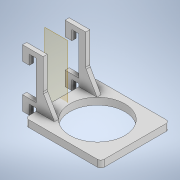
# Autodesk Inventor part: round_2_0_inchHoleV01
Saved by Autodesk Inventor 2021 (Build 250183000, 183)
## iProperties
Created: 2020-03-07
Part Number: round_2_0_inchHoleV01
Material: Generic
Document SubType Name: Modeling
Designer: robst
Density: 1 g/cm^3
Appearance: Default
Author: robst
Autodesk Inventor part; units mm, degrees
ref_plane "YZ Plane" through (0, 0, 0) normal (1, 0, 0) x (0, 1, 0)
ref_plane "XZ Plane" through (0, 0, 0) normal (0, 1, 0) x (-1, 0, 0)
sketch "Sketch1" plane through (0, 0, 0) normal (0, 0, 1) x (1, 0, 0)
  line L0 (0, 6.35) -> (0, 53.34)
  line L1 (0, 53.34) -> (-19.05, 53.34)
  line L2 (-19.05, 53.34) -> (-19.05, 55.245)
  line L3 (-12.7, 48.895) -> (-6.35, 48.895)
  line L4 (-6.35, 48.895) -> (-6.35, 13.335)
  line L5 (-6.35, 13.335) -> (-19.05, 13.335)
  line L6 (-19.05, 13.335) -> (-19.05, 12.7)
  line L7 (-12.7, 8.89) -> (-6.35, 8.89)
  line L8 (-6.35, 8.89) -> (-6.35, 0)
  line L9 (-6.35, 0) -> (0, 0)
  line L10 (-19.05, 55.245) -> (-19.05, 40.005)
  line L11 (-19.05, 40.005) -> (-12.7, 40.005)
  line L12 (-12.7, 40.005) -> (-12.7, 48.895)
  line L13 (-19.05, 12.7) -> (-19.05, 0)
  line L14 (-19.05, 0) -> (-12.7, 0)
  line L15 (-12.7, 0) -> (-12.7, 8.89)
  line L16 (0, 0) -> (0, 6.35)
  line L17 (0, 0) -> (10.16, 0)
  line L18 (10.16, 0) -> (0, 23.7508)
  point P0 (-19.05, 53.34)
  point P1 (-19.05, 11.43)
  dimension "d1" = 35.56
  dimension "d2" = 4.445
  dimension "d3" = 4.445
  dimension "d4" = 6.35
  dimension "d6" = 6.35
  dimension "d7" = 6.35
  dimension "d13" = 13.335
  dimension "d14" = 13.335
  dimension "d35" = 10.16
  dimension "d36" = 66.84
  constraints: 38 end point, 9 perpendicular, 5 point on line, 3 vertical, 1 collinear, 1 horizontal, 1 parallel
  measures "d1" distance of L3.end L4.end
  measures "d2" distance between parallel lines of L5 L7
  measures "d3" distance between parallel lines of L1 L3
  measures "d4" distance between parallel lines of L4 L0
  measures "d6" distance between parallel lines of L12 L4
  measures "d7" distance between parallel lines of L10 L12
  measures "d13" distance between parallel lines of L11 L1
  measures "d14" distance between parallel lines of L5 L14
  measures "d35" distance of L9.end L17.end
  measures "d36" angle of L18 L17
extrude "Extrusion1" add sketch "Sketch1" along normal mid plane 3.81 contours L16 L9 L8 L7 L15 L14 L13 L6 L5 L4 L3 L12 L11 L10 L1 L0
ref_plane "Work Plane1" through (0, 0, 19.685) normal (0, 0, 1) x (1, 0, 0)
mirror "Mirror1" about plane through (0, 0, 19.685) normal (0, 0, 1) of "Extrusion1"
sketch "Sketch4" plane through (0, 0, 19.685) normal (0, 0, 1) x (1, 0, 0)
  line L0 (-6.35, 8.89) -> (-6.35, 0) projected
  line L1 (-6.35, 0) -> (63.5, 0)
  line L2 (63.5, 0) -> (63.5, 6.35)
  line L3 (63.5, 6.35) -> (-6.35, 6.35)
  line L4 (-6.35, 6.35) -> (-6.35, 0)
  point P0 (0, 0)
  dimension "d23" = 69.85
  dimension "d24" = 6.35
  constraints: 8 end point, 2 parallel, 1 horizontal, 1 perpendicular
  measures "d23" distance of L3.end L2.end
  measures "d24" distance of L2.end L1.end
extrude "Extrusion4" add sketch "Sketch4" along normal mid plane 63.5
sketch "Sketch5" plane through (-6.35, 6.35, 51.435) normal (0, 1, 0) x (1, 0, 0)
  line L0 (0, 63.5) -> (69.85, 63.5) construction
  line L1 (69.85, 63.5) -> (69.85, 0) construction
  line L2 (0, 0) -> (69.85, 0) construction
  line L3 (0, 0) -> (0, 63.5) construction
  line L4 (0, 63.5) -> (69.85, 0) construction
  line L5 (69.85, 63.5) -> (0, 0) construction
  circle A0 centre (34.925, 31.75) radius 25.4
  point P0 (6.35, 51.435)
  dimension "d32" = 50.8
  constraints: 4 end point, 1 centre point, 1 midpoint
  measures "d32" diameter of A0
fillet "Fillet1" radius 3.175 4 edges at (-6.35, 3.175, 51.435) (63.5, 3.175, 51.435) (63.5, 3.175, -12.065) (-6.35, 3.175, -12.065)
extrude "Extrusion6" cut sketch "Sketch5" against normal through all
sketch "Sketch6" plane through (0, 0, 1.905) normal (0, 0, 1) x (1, 0, 0)
  line L0 (-3.175, 6.35) -> (60.325, 6.35) projected
  line L1 (10.4354, 6.35) -> (0, 6.35)
  line L2 (10.4354, 6.35) -> (1.4968, 21.8321)
  line L3 (10.4354, 6.35) -> (28.3126, 6.35) construction
  line L4 (1.4968, 21.8321) -> (0, 24.4246)
  line L5 (0, 53.34) -> (0, 6.35) projected
  line L6 (0, 24.4246) -> (0, 6.35)
  point P0 (0, 0)
  dimension "d37" = 120
  constraints: 10 end point, 4 point on line, 1 equal length, 1 horizontal, 1 perpendicular
  measures "d37" angle of L3 L2
extrude "Extrusion7" add sketch "Sketch6" against normal blind 3.81
mirror "Mirror2" about plane through (0, 0, 19.685) normal (0, 0, 1) of "Extrusion7"
fillet "Fillet2" radius 3.175 2 edges at (0, 24.4246, 39.37) (0, 24.4246, 0)
equation "\"d11\" = width"
equation "\"d15\" = oneHalfSpacing"
equation "\"width\" = 3.81"
equation "\"spacing\" = 39.37"
equation "\"oneHalfSpacing\" = 0.5 * spacing"
body "Solid1"
